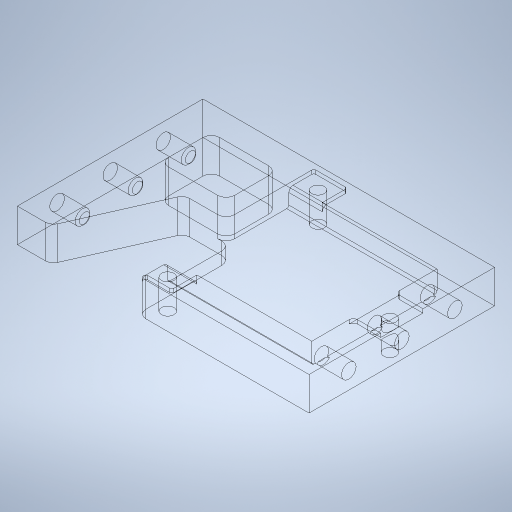
# Autodesk Inventor part: Servo Support
Saved by Autodesk Inventor 2023.2 (Build 272271000, 271)
## iProperties
Created: 2024-01-22
Part Number: Servo Support
Material: Nylon 6/6
Document SubType Name: Modeling
Designer: Nathan Cai
Density: 1.13 g/cm^3
Appearance: Nylon 6
Author: Nathan Cai
Autodesk Inventor part; units mm, degrees
ref_plane "YZ Plane" through (0, 0, 0) normal (1, 0, 0) x (0, 1, 0)
ref_plane "XZ Plane" through (0, 0, 0) normal (0, 1, 0) x (-1, 0, 0)
ref_plane "XY Plane" through (0, 0, 0) normal (0, 0, 1) x (1, 0, 0)
sketch "Sketch1" plane through (0, 0, 0) normal (0, 1, 0) x (-1, 0, 0)
  line L0 (-17.75, 15) -> (17.75, 15)
  line L1 (17.75, 15) -> (17.75, -15)
  line L2 (17.75, -15) -> (-17.75, -15)
  line L3 (-17.75, -15) -> (-17.75, 15)
  line L4 (-17.75, 15) -> (17.75, -15) construction
  line L5 (17.75, 15) -> (-17.75, -15) construction
  line L6 (17.75, 0) -> (-17.75, 0) construction
  line L7 (17.75, 21) -> (9.75, 21)
  line L8 (9.75, 21) -> (9.75, -21)
  line L9 (9.75, -21) -> (17.75, -21)
  line L10 (17.75, -21) -> (17.75, 21)
  line L11 (17.75, 21) -> (9.75, -21) construction
  line L12 (9.75, 21) -> (17.75, -21) construction
  line L13 (13.75, 21) -> (13.75, -21) construction
  circle A0 centre (13.75, -18) radius 1.5
  line L14 (-17.75, 5.05) -> (-24.15, 5.05)
  line L15 (-24.15, 5.05) -> (-24.15, -5.05) construction
  line L16 (-24.15, -5.05) -> (-17.75, -5.05)
  line L17 (-17.75, -5.05) -> (-17.75, 5.05)
  line L18 (-17.75, 5.05) -> (-24.15, -5.05) construction
  line L19 (-24.15, 5.05) -> (-17.75, -5.05) construction
  circle A1 centre (-21.45, 0) radius 1.5
  circle A2 centre (13.75, 18) radius 1.5
  line L20 (17.75, 10.9) -> (21.05, 10.9)
  line L21 (21.05, 10.9) -> (21.05, 5.9)
  line L22 (21.05, 5.9) -> (17.75, 5.9)
  line L23 (17.75, 5.9) -> (17.75, 10.9)
  line L24 (-24.3188, 22.225) -> (45.5312, 22.225)
  line L25 (45.5312, 22.225) -> (45.5312, -22.225)
  line L26 (45.5312, -22.225) -> (-24.3188, -22.225)
  line L27 (-24.3188, -22.225) -> (-24.3188, 22.225)
  line L28 (-24.3188, 22.225) -> (45.5312, -22.225) construction
  line L29 (45.5312, 22.225) -> (-24.3188, -22.225) construction
  line L30 (21.05, 8.4) -> (17.75, 8.4) construction
  line L31 (25.6875, 15.4) -> (17.75, 15.4)
  line L32 (17.75, 15.4) -> (17.75, 1.4)
  line L33 (17.75, 1.4) -> (25.6875, 1.4)
  line L34 (25.6875, 1.4) -> (25.6875, 15.4)
  line L35 (25.6875, 15.4) -> (17.75, 1.4) construction
  line L36 (17.75, 15.4) -> (25.6875, 1.4) construction
  line L37 (17.75, 0) -> (27.75, 0)
  line L38 (27.75, 0) -> (27.75, 22.225)
  line L39 (27.75, 22.225) -> (17.75, 22.225)
  line L40 (17.75, 22.225) -> (17.75, 0)
  line L41 (-17.75, -5.05) -> (-24.3188, -5.05)
  line L42 (-24.3188, -5.05) -> (-24.3188, 5.05)
  line L43 (-24.3188, 5.05) -> (-17.75, 5.05)
  line L44 (-17.75, 5.05) -> (-17.75, -5.05)
  line L45 (37.5312, -16.225) -> (21.75, -16.225)
  line L46 (21.75, -16.225) -> (21.75, -4)
  line L47 (21.75, -4) -> (37.5312, -4)
  line L48 (37.5312, -4) -> (37.5312, -16.225)
  line L49 (27.75, 0) -> (37.5312, 22.225)
  point P0 (0, 0)
  point P1 (13.75, 0)
  point P2 (-20.95, 0)
  point P3 (10.6062, 0)
  point P4 (21.7187, 8.4)
  point P5 (17.75, 15)
  dimension "d0" = 35.5
  dimension "d1" = 30
  dimension "d2" = 8
  dimension "d3" = 42
  dimension "d4" = 3
  dimension "d5" = 18
  dimension "d7" = 10.1
  dimension "d8" = 3
  dimension "d9" = 35.2
  dimension "d10" = 41.9
  dimension "d11" = 5
  dimension "d12" = 45.2
  dimension "d13" = 9.6
  dimension "d14" = 69.85
  dimension "d15" = 27.7812
  dimension "d16" = 44.45
  dimension "d17" = 7.9375
  dimension "d18" = 14
  dimension "d19" = 10
  dimension "d50" = 8
  dimension "d51" = 4
  dimension "d52" = 6
  dimension "d53" = 4
  dimension "d54" = 8
  constraints: 100 end point, 18 parallel, 16 midpoint, 14 point on line, 9 horizontal, 9 perpendicular, 3 centre point, 1 symmetric about line, 1 other
  measures "d0" distance of L1.end L2.end
  measures "d1" distance between parallel lines of L0 L2
  measures "d2" distance of L9.end L8.end
  measures "d3" distance of L8.end L7.end
  measures "d4" diameter of A0
  measures "d5" distance from line of A0.centre L6
  measures "d7" distance of L15.end L14.end
  measures "d8" diameter of A1
  measures "d9" distance from line of L13 A1.centre
  measures "d10" distance between parallel lines of L15 L10
  measures "d11" distance between parallel lines of L20 L22
  measures "d12" distance between parallel lines of L15 L21
  measures "d13" vertical distance of A2.centre L30.start
  measures "d14" distance of L25.end L26.end
  measures "d15" distance between parallel lines of L25 L1
  measures "d16" distance between parallel lines of L24 L26
  measures "d17" distance of L33.end L32.end
  measures "d18" distance of L32.end L31.end
  measures "d19" distance between parallel lines of L1 L38
  measures "d50" distance between parallel lines of L25 L48
  measures "d51" distance between parallel lines of L1 L46
  measures "d52" distance between parallel lines of L26 L45
  measures "d53" distance between parallel lines of L37 L47
  measures "d54" distance from line of L25 L49.end
extrude "Extrusion1" add sketch "Sketch1" against normal blind 8 contours L3 L14 L43 L27 L24 L40 L7 L8 L0 | L0 L8 L2 L3 | L8 L7 L10 L0 | L0 L1 L2 L8 | L3 L16 L41 L27 L43 L14 | L10 L31 L34 L33 L1 L22 L21 L20 | L8 L9 L10 L1 L37 L49 L24 L25 L26 L27 L41 L16 L3 L2 | L2 L10 L9 L8 | L20 L21 L22 L1 | L10 L40 L24 L38 L37 L1 L33 L34 L31 | L24 L49 L38 | A0 | A1 | A2 | L45 L46 L47 L48
extrude "Extrusion2" cut sketch "Sketch1" against normal through all contours L10 L31 L34 L33 L1 L22 L21 L20 | L20 L21 L22 L1 | L10 L40 L24 L38 L37 L1 L33 L34 L31 | L24 L49 L38 | L45 L46 L47 L48
extrude "Extrusion3" cut sketch "Sketch1" against normal blind 5 contours L0 L8 L2 L3 | L0 L1 L2 L8
extrude "Extrusion4" cut sketch "Sketch1" against normal blind 0.9 contours L8 L7 L10 L0 | L0 L1 L2 L8 | L3 L16 L41 L27 L43 L14 | L2 L10 L9 L8 | A0 | A1 | A2
extrude "Extrusion5" cut sketch "Sketch1" against normal through all contours A0 | A1 | A2
thicken "Thicken1" operation cut thickness 1 both sides no extend neighbours no toward (1, 0, 0) faces at (-17.75, -7, 12.4083)
fillet "Fillet4" radius 2 9 edges at (-17.75, -2.5, 0) (-16.75, -6.5, 0) (-27.75, -4, 0) (-16.75, -4, 22.225) (-37.5312, -4, 22.225) (-37.5312, -4, -16.225) (-21.75, -4, -16.225) (-21.75, -4, -4) (-37.5312, -4, -4)
fillet "Fillet1" radius 0.5 6 edges at (0, -5, -15) (0.5, -5, 15) (-17.75, -0.45, -21) (-9.75, -0.45, -21) (-9.75, -0.45, 21) (-16.5937, -0.45, 21)
fillet "Fillet2" radius 1 4 edges at (-13.75, -0.9, -15) (-13.25, -0.9, 15) (17.75, -0.45, -5.05) (17.75, -0.45, 5.05)
ref_plane "Work Plane1" through (-10.6062, -8, 22.225) normal (1, 0, 0) x (0, 0, -1)
sketch "Sketch2" plane through (24.3188, -8, 22.225) normal (1, 0, 0) x (0, 0, -1)
  line L0 (44.45, 8) -> (44.45, 0) projected
  line L1 (44.45, 4) -> (0, 4) construction
  line L2 (0, 8) -> (0, 0) projected
  circle A0 centre (34.925, 4) radius 1.7526
  circle A1 centre (22.225, 4) radius 1.7526
  circle A2 centre (9.525, 4) radius 1.7526
  point P0 (22.225, 8)
  dimension "d36" = 3.5052
  dimension "d39" = 12.7
  dimension "d44" = 9.525
  constraints: 3 centre point, 2 end point, 2 midpoint, 1 horizontal, 1 point on line, 4 other
  measures "d36" diameter of A0
  measures "d39" distance of A0.centre A1.centre
  measures "d44" distance from line of L0 A0.centre
extrude "Extrusion6" cut sketch "Sketch2" against normal up to surface (6.5688 mm away)
chamfer "Chamfer1" distance 0.5 angle 45 3 edges at (17.75, -5.7526, -12.7) (17.75, -5.7526, 0) (17.75, -5.7526, 12.7)
mirror "Mirror1" about plane through (-10.6062, -8, 22.225) normal (1, 0, 0) of "Extrusion6", "Chamfer1"
body "Solid1"
